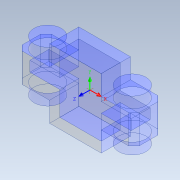
# Autodesk Inventor part: body_inventor
Saved by Autodesk Inventor 2020 (Build 240168000, 168)
## iProperties
Created: 2021-01-07
Part Number: body_inventor
Material: Generic
Document SubType Name: Modeling
Designer: DELL
Density: 1 g/cm^3
Appearance: Clear - Blue
Author: DELL
Autodesk Inventor part; units mm, degrees
ref_plane "YZ Plane" through (0, 0, 0) normal (1, 0, 0) x (0, 1, 0)
ref_plane "XZ Plane" through (0, 0, 0) normal (0, 1, 0) x (-1, 0, 0)
ref_plane "XY Plane" through (0, 0, 0) normal (0, 0, 1) x (1, 0, 0)
sketch "Sketch4" plane through (0, 0, 0) normal (0, 0, 1) x (1, 0, 0)
  line L0 (75, -100) -> (-75, -100)
  line L1 (-75, -100) -> (-75, 100)
  line L2 (-75, 100) -> (75, 100)
  line L3 (75, 100) -> (75, -100)
  line L4 (75, -100) -> (-75, 100) construction
  line L5 (-75, -100) -> (75, 100) construction
  line L6 (170, -42) -> (-170, -42)
  line L7 (-170, -42) -> (-170, 42)
  line L8 (-170, 42) -> (170, 42)
  line L9 (170, 42) -> (170, -42)
  line L10 (170, -42) -> (-170, 42) construction
  line L11 (-170, -42) -> (170, 42) construction
  point P0 (0, 0)
  point P1 (0, 0)
  point P2 (0, 0)
  point P3 (75, 42)
  point P4 (-75, 42)
  point P5 (-75, -42)
  point P6 (75, -42)
  dimension "d17" = 84
  dimension "d18" = 340
  dimension "d19" = 150
  dimension "d20" = 200
  constraints: 24 end point, 5 midpoint, 4 parallel, 2 horizontal, 2 perpendicular, 1 coincident
  measures "d17" distance of L8.end L6.start
  measures "d18" distance of L6.start L6.end
  measures "d19" distance of L0.start L0.end
  measures "d20" distance of L2.end L0.start
extrude "Extrusion4" add sketch "Sketch4" along normal mid plane 85
sketch "Sketch5" plane through (0, 0, 0) normal (0, 1, 0) x (-1, 0, 0)
  circle A0 centre (-123, 0) radius 39.5
  circle A1 centre (123, 0) radius 39.5
  line L0 (75, 42.5) -> (-75, 42.5) construction
  line L1 (0, 42.5) -> (0, -42.5) construction
  line L2 (-75, -42.5) -> (75, -42.5) construction
  line L3 (-170, -42.5) -> (-170, 42.5) construction
  line L4 (-170, 0) -> (170, 0) construction
  line L5 (170, -42.5) -> (170, 42.5) construction
  circle A2 centre (-123, 0) radius 31.5
  circle A3 centre (123, 0) radius 31.5
  line L6 (-155, 42.5) -> (-170, 27.5)
  line L7 (-170, -27.5) -> (-155, -42.5)
  line L8 (-170, -42.5) -> (-75, -42.5) projected
  line L9 (170, 42.5) -> (75, 42.5) projected
  line L10 (155, 42.5) -> (170, 27.5)
  line L11 (170, -27.5) -> (155, -42.5)
  line L12 (-75, 42.5) -> (-170, 42.5) projected
  line L13 (75, -42.5) -> (170, -42.5) projected
  line L14 (-170, 42.5) -> (-170, -42.5)
  line L15 (170, 42.5) -> (170, -42.5)
  point P0 (0, 0)
  point P1 (-170, -27.5)
  dimension "d23" = 79
  dimension "d24" = 246
  dimension "d39" = 63
  dimension "d42" = 15
  dimension "d43" = 45
  constraints: 16 end point, 9 point on line, 5 perpendicular, 4 centre point, 4 midpoint, 3 equal length, 2 coincident, 2 equal radius, 1 symmetric about line
  measures "d23" diameter of A0
  measures "d24" distance of A1.centre A0.centre
  measures "d39" diameter of A2
  measures "d42" distance of L3.end L6.end
  measures "d43" angle of L6 L3
extrude "Extrusion5" add sketch "Sketch5" against normal blind 32 from surface at -42 contours A0 | A1 | A2 | A3
sketch "Sketch6" plane through (0, 0, 0) normal (0, 0, 1) x (1, 0, 0)
  line L0 (147, 15) -> (-147, 15)
  line L1 (-147, 15) -> (-147, -15)
  line L2 (-147, -15) -> (147, -15)
  line L3 (147, -15) -> (147, 15)
  line L4 (147, 15) -> (-147, -15) construction
  line L5 (-147, 15) -> (147, -15) construction
  line L6 (-60, 85) -> (60, 85)
  line L7 (60, 85) -> (60, -85)
  line L8 (60, -85) -> (-60, -85)
  line L9 (-60, -85) -> (-60, 85)
  line L10 (-60, 85) -> (60, -85) construction
  line L11 (60, 85) -> (-60, -85) construction
  line L12 (75, -100) -> (-75, -100) projected
  line L13 (-75, 42) -> (-75, 100) projected
  line L14 (-170, -42) -> (-170, 42) projected
  line L15 (-75, -42) -> (-170, -42) projected
  point P0 (0, 0)
  point P1 (-60, -15)
  point P2 (60, -15)
  point P3 (60, 15)
  point P4 (-60, 15)
  dimension "d27" = 15
  dimension "d28" = 15
  dimension "d29" = 23
  dimension "d30" = 27
  dimension "d46" = 30
  constraints: 24 end point, 4 midpoint, 4 parallel, 2 horizontal, 2 perpendicular
  measures "d27" distance between parallel lines of L12 L8
  measures "d28" distance between parallel lines of L13 L9
  measures "d29" distance between parallel lines of L14 L1
  measures "d30" distance between parallel lines of L15 L2
  measures "d46" distance between parallel lines of L2 L0
extrude "Extrusion6" cut sketch "Sketch6" along normal mid plane 55
extrude "Extrusion8" cut sketch "Sketch5" against normal through all both and the other way through all contours L7 L8 L14 | L6 L14 L12 | L15 L10 L9 | L15 L13 L11
mirror "Mirror1" about plane through (0, 0, 0) normal (0, 1, 0) of "Extrusion5"
equation "\"d21\" = body_thickness"
equation "\"d27\" = wall_thickness"
equation "\"d28\" = wall_thickness"
equation "\"d31\" = body_thickness - 2 * wall_thickness"
equation "\"wall_thickness\" = 15"
equation "\"body_thickness\" = 85"
body "Solid1"
body "Solid2"
